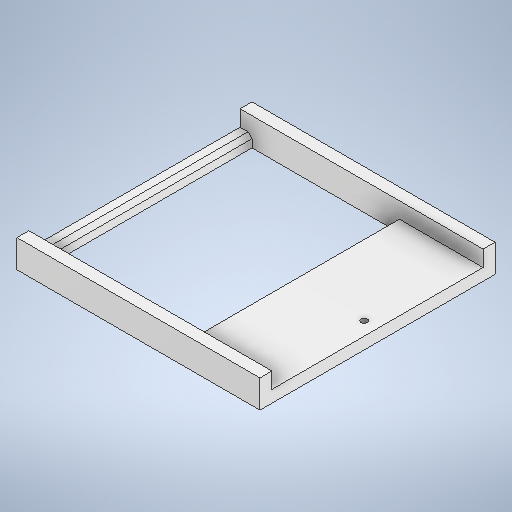
# Autodesk Inventor part: Module Holder V1
Saved by Autodesk Inventor 2025 (Build 290162000, 162)
## iProperties
Created: 2024-03-20
Part Number: Module Holder V1
Material: ABS Plastic
Document SubType Name: Modeling
Designer: cfang
Density: 1.06 g/cm^3
Appearance: Smooth - White
Author: cfang
Autodesk Inventor part; units mm, degrees
ref_plane "YZ Plane" through (0, 0, 0) normal (1, 0, 0) x (0, 1, 0)
ref_plane "XZ Plane" through (0, 0, 0) normal (0, 1, 0) x (-1, 0, 0)
ref_plane "XY Plane" through (0, 0, 0) normal (0, 0, 1) x (1, 0, 0)
sketch "Sketch1" plane through (0, 0, 0) normal (0, 1, 0) x (-1, 0, 0)
  line L0 (-30.5, -29.5) -> (30.5, -29.5)
  line L1 (30.5, -29.5) -> (30.5, 29.5)
  line L2 (30.5, 29.5) -> (-30.5, 29.5)
  line L3 (-30.5, 29.5) -> (-30.5, -29.5)
  line L4 (-30.5, -29.5) -> (30.5, 29.5) construction
  line L5 (30.5, -29.5) -> (-30.5, 29.5) construction
  point P0 (0, 0)
  dimension "d0" = 59
  dimension "d1" = 61
  constraints: 12 end point, 2 midpoint, 2 parallel, 1 horizontal, 1 perpendicular
  measures "d0" distance of L0.end L1.end
  measures "d1" distance of L1.end L2.end
extrude "Extrusion1" add sketch "Sketch1" along normal blind 7
sketch "Sketch2" plane through (0, 7, 0) normal (0, 1, 0) x (1, 0, 0)
  line L0 (-30.5, 29.5) -> (-30.5, -29.5) projected
  line L1 (30.5, 26.5) -> (-30.5, 26.5)
  line L2 (-30.5, 26.5) -> (-30.5, -26.5)
  line L3 (-30.5, -26.5) -> (30.5, -26.5)
  line L4 (30.5, -26.5) -> (30.5, 26.5)
  line L5 (30.5, 26.5) -> (-30.5, -26.5) construction
  line L6 (-30.5, 26.5) -> (30.5, -26.5) construction
  point P0 (0, 0)
  point P1 (-30.5, 26.5)
  dimension "d4" = 53
  constraints: 12 end point, 2 midpoint, 2 parallel, 1 horizontal, 1 perpendicular, 1 point on line
  measures "d4" distance between parallel lines of L3 L1
extrude "Extrusion2" cut sketch "Sketch2" against normal blind 4
sketch "Sketch3" plane through (0, 3, 0) normal (0, 1, 0) x (1, 0, 0)
  point P0 (0, 0)
  point P1 (27.15, 0)
  dimension "d8" = 27.15
  measures "d8" distance of point (0, 0) point (27.15, 0)
hole "Hole1" at (27.15, 3, 0) direction (0, -1, 0) diameter 1.567 end through all thread size "M2x0.4" class "6H" standard "ANSI Metric M Profile"
sketch "Sketch4" plane through (0, 3, 0) normal (0, 1, 0) x (1, 0, 0)
  line L0 (30.5, -26.5) -> (-30.5, -26.5) projected
  line L1 (-27.5, 26.5) -> (9.5, 26.5)
  line L2 (9.5, 26.5) -> (9.5, -26.5)
  line L3 (9.5, -26.5) -> (-27.5, -26.5)
  line L4 (-27.5, -26.5) -> (-27.5, 26.5)
  line L5 (-30.5, 26.5) -> (30.5, 26.5) projected
  line L6 (-30.5, -26.5) -> (-30.5, 26.5) projected
  point P0 (0, 0)
  dimension "d16" = 37
  dimension "d19" = 3
  constraints: 8 end point, 2 parallel, 2 point on line, 1 horizontal, 1 perpendicular
  measures "d16" distance of L2.end L3.end
  measures "d19" distance between parallel lines of L6 L4
extrude "Extrusion3" cut sketch "Sketch4" against normal through all contours L0 L4 L1 L2
chamfer "Chamfer1" distance 1 angle 45 1 edges at (-27.5, 3, 0)
equation "\"d8\" = d7"
equation "\"d7\" = 27.15"
body "Solid1"
